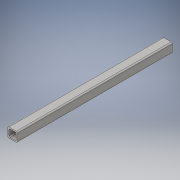
# Autodesk Inventor part: 2ndVert
Saved by Autodesk Inventor 2016 (Build 200138000, 138)
## iProperties
Created: 2016-06-23
Part Number: 2ndVert
Material: Generic
Document SubType Name: Modeling
Designer: cutrones
Density: 1 g/cm^3
Appearance: Default
Author: cutrones
Autodesk Inventor part; units mm, degrees
ref_plane "YZ Plane" through (0, 0, 0) normal (1, 0, 0) x (0, 1, 0)
ref_plane "XZ Plane" through (0, 0, 0) normal (0, 1, 0) x (-1, 0, 0)
ref_plane "XY Plane" through (0, 0, 0) normal (0, 0, 1) x (1, 0, 0)
sketch "Sketch1" plane through (0, 0, 0) normal (0, 0, 1) x (1, 0, 0)
  line L0 (3.175, 0) -> (22.225, 0)
  line L1 (25.4, 3.175) -> (25.4, 22.225)
  line L2 (22.225, 25.4) -> (3.175, 25.4)
  line L3 (0, 22.225) -> (0, 3.175)
  arc A0 (3.175, 25.4) -> (0, 22.225) centre (3.175, 22.225) ccw
  arc A1 (25.4, 22.225) -> (22.225, 25.4) centre (22.225, 22.225) ccw
  arc A2 (22.225, 0) -> (25.4, 3.175) centre (22.225, 3.175) ccw
  arc A3 (0, 3.175) -> (3.175, 0) centre (3.175, 3.175) ccw
  line L4 (6.35, 3.175) -> (19.05, 3.175)
  line L5 (22.225, 6.35) -> (22.225, 19.05)
  line L6 (19.05, 22.225) -> (6.35, 22.225)
  line L7 (3.175, 19.05) -> (3.175, 6.35)
  arc A4 (6.35, 22.225) -> (3.175, 19.05) centre (6.35, 19.05) ccw
  arc A5 (19.05, 3.175) -> (22.225, 6.35) centre (19.05, 6.35) ccw
  arc A6 (22.225, 19.05) -> (19.05, 22.225) centre (19.05, 19.05) ccw
  arc A7 (3.175, 6.35) -> (6.35, 3.175) centre (6.35, 6.35) ccw
  point P0 (0, 0)
  point P1 (25.4, 25.4)
  point P2 (25.4, 0)
  point P3 (0, 25.4)
  dimension "d0" = 25.4
  dimension "d1" = 25.4
  dimension "d2" = 3.175
  dimension "d3" = 3.175
  constraints: 16 end point, 16 point on circle, 16 tangent, 12 point on line, 8 centre point, 6 equal radius, 4 parallel, 2 horizontal, 2 perpendicular
  measures "d0" distance of point (0, 25.4) point (25.4, 25.4)
  measures "d1" distance of point (25.4, 25.4) point (25.4, 0)
  measures "d2" radius of A0
  measures "d3" radius of A4
extrude "Extrusion1" add sketch "Sketch1" along normal blind 406.4
body "Solid1"
